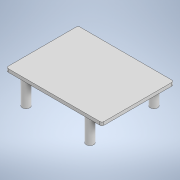
# Autodesk Inventor part: sliding_surface
Saved by Autodesk Inventor 2022 (Build 260153000, 153)
## iProperties
Created: 2021-07-07
Part Number: sliding_surface
Material: Generic
Document SubType Name: Modeling
Designer: fraaw
Density: 1 g/cm^3
Appearance: Default
Author: fraaw
## iProperties of the stored document sliding_surface_3DPrint.ipt
Created: 2021-07-07
Part Number: sliding_surface_3DPrint
Material: Generic
Document SubType Name: Modeling
Designer: fraaw
Density: 1 g/cm^3
Appearance: Default
Author: fraaw
Autodesk Inventor part; units mm, degrees
ref_plane "YZ Plane" through (0, 0, 0) normal (1, 0, 0) x (0, 1, 0)
ref_plane "XZ Plane" through (0, 0, 0) normal (0, 1, 0) x (-1, 0, 0)
ref_plane "XY Plane" through (0, 0, 0) normal (0, 0, 1) x (1, 0, 0)
sketch "Sketch2" plane through (0, 0, 0) normal (0, 1, 0) x (-1, 0, 0)
  line L0 (-60, 60) -> (60, 60)
  line L1 (60, 60) -> (60, -60)
  line L2 (60, -60) -> (-60, -60)
  line L3 (-60, -60) -> (-60, 60)
  line L4 (-60, 60) -> (60, -60) construction
  line L5 (60, 60) -> (-60, -60) construction
  point P0 (0, 0)
  dimension "d4" = 120
  dimension "d5" = 120
  constraints: 12 end point, 2 midpoint, 2 parallel, 1 horizontal, 1 perpendicular
  measures "d4" distance of L0.end L1.end
  measures "d5" distance of L0.start L0.end
extrude "Extrusion2" add sketch "Sketch2" along normal blind 4
sketch "Sketch3" plane through (0, 0, 0) normal (0, -1, 0) x (1, 0, 0)
  line L0 (-40, 40) -> (40, 40) construction
  line L1 (40, 40) -> (40, -40) construction
  line L2 (40, -40) -> (-40, -40) construction
  line L3 (-40, -40) -> (-40, 40) construction
  line L4 (-40, 40) -> (40, -40) construction
  line L5 (40, 40) -> (-40, -40) construction
  circle A0 centre (40, 40) radius 4.7
  circle A1 centre (-40, 40) radius 4.7
  circle A2 centre (-40, -40) radius 4.7
  circle A3 centre (40, -40) radius 4.7
  point P0 (0, 0)
  dimension "d8" = 80
  dimension "d9" = 80
  dimension "d10" = 9.4
  dimension "d13" = 360
  constraints: 12 end point, 4 centre point, 2 midpoint, 2 parallel, 1 coincident, 1 horizontal, 1 perpendicular, 9 other
  measures "d8" distance of L0.end L1.end
  measures "d9" distance of L0.start L0.end
  measures "d10" diameter of A0
extrude "Extrusion3" add sketch "Sketch3" along normal blind 30
sketch "Sketch4" plane through (0, 0, 0) normal (0, -1, 0) x (1, 0, 0)
  point P0 (0, 0)
  point P1 (0, 0)
  constraints: 1 coincident
hole "Hole1" at (0, 0, 0) direction (0, 1, 0) diameter 16 depth 1
sketch "Sketch5" plane through (0, 4, 0) normal (0, 1, 0) x (1, 0, 0)
  line L0 (60, -60) -> (60, 60) projected
  line L1 (-60, -60) -> (60, -60)
  line L2 (60, -60) -> (60, -45)
  line L3 (60, -45) -> (-60, -45)
  line L4 (-60, -45) -> (-60, -60)
  line L5 (60, 60) -> (-60, 60) projected
  line L6 (-60, 60) -> (60, 60)
  line L7 (60, 60) -> (60, 45)
  line L8 (60, 45) -> (-60, 45)
  line L9 (-60, 45) -> (-60, 60)
  point P0 (0, 0)
  dimension "d24" = 15
  dimension "d25" = 15
  constraints: 16 end point, 4 parallel, 2 horizontal, 2 perpendicular, 2 point on line
  measures "d24" distance of L3.end L1.start
  measures "d25" distance of L8.end L5.end
extrude "Extrusion4" cut sketch "Sketch5" against normal up to surface (4 mm away)
fillet "Fillet2" radius 2.5 4 edges at (60, 2, 45) (60, 2, -45) (-60, 2, 45) (-60, 2, -45)
body "Solid2"
